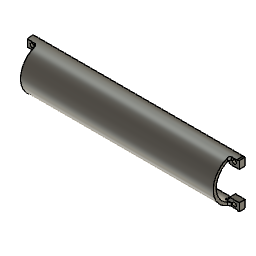
Cache cable (Autodesk Fusion 360 design; units mm, degrees)
Autodesk Fusion 360 part; units mm, degrees
sketch "Esquisse1" plane through (0, 0, 0) normal (1, 0, 0) x (0, 1, 0)
  circle A0 centre (0, 10) radius 10
  circle A1 centre (0, 10) radius 11.5
  line L0 (0, -1.5) -> (0, 21.5)
  dimension "d1" = 20
  dimension "d2" = 23
  constraint coincident origin A0
  constraint concentric A0 A1
  constraint coincident A1 L0.start
  constraint coincident A1 L0.end
  constraint vertical L0
  measures "d1" diameter of A0
  measures "d2" diameter of A1
extrude "Extrusion1" add sketch "Esquisse1" against normal blind 100 contours A0 A1 L0 picked at (-1.0681, 20.92)
sketch "Esquisse2" plane through (0, 0, 0) normal (0, 1, 0) x (1, 0, 0)
  line L0 (0, -21.5) -> (5, -21.5)
  line L1 (5, -21.5) -> (5, -17.5)
  line L2 (5, -17.5) -> (0, -17.5)
  line L3 (0, -17.5) -> (0, -21.5)
  line L4 (0, 1.5) -> (5, 1.5)
  line L5 (5, 1.5) -> (5, -2.5)
  line L6 (5, -2.5) -> (0, -2.5)
  line L7 (0, -2.5) -> (0, 1.5)
  circle A0 centre (2.5, -19.5) radius 1
  circle A1 centre (2.5, -0.5) radius 1
  line L8 (-100, -17.5) -> (-105, -17.5)
  line L9 (-105, -17.5) -> (-105, -21.5)
  line L10 (-105, -21.5) -> (-100, -21.5)
  line L11 (-100, -21.5) -> (-100, -17.5)
  line L12 (-100, 1.5) -> (-105, 1.5)
  line L13 (-105, 1.5) -> (-105, -2.5)
  line L14 (-105, -2.5) -> (-100, -2.5)
  line L15 (-100, -2.5) -> (-100, 1.5)
  circle A2 centre (-102.5, -19.5) radius 1
  circle A3 centre (-102.5, -0.5) radius 1
  dimension "d5" = 1.5
  dimension "d6" = 21.5
  dimension "d9" = 4
  dimension "d10" = 4
  dimension "d11" = 2
  dimension "d12" = 2
  dimension "d13" = 2.5
  dimension "d14" = 2
  dimension "d15" = 5
  dimension "d16" = 2.5
  dimension "d17" = 2
  dimension "d24" = 100
  dimension "d25" = 100
  dimension "d26" = 1.5
  dimension "d27" = 23
  dimension "d28" = 4
  dimension "d29" = 4
  dimension "d30" = 5
  dimension "d31" = 5
  dimension "d32" = 2
  dimension "d33" = 2
  dimension "d34" = 2.5
  dimension "d35" = 2
  dimension "d36" = 2.5
  dimension "d37" = 2
  constraint horizontal L0
  constraint vertical L1
  constraint horizontal L2
  constraint vertical L3
  constraint horizontal L4
  constraint vertical L5
  constraint horizontal L6
  constraint vertical L7
  constraint horizontal L8
  constraint vertical L9
  constraint horizontal L10
  constraint vertical L11
  constraint horizontal L12
  constraint vertical L13
  constraint horizontal L14
  constraint vertical L15
  measures "d5" distance of origin L4
  measures "d6" distance of origin L0
  measures "d9" distance of L4.end L5.end
  measures "d10" distance of L0.end L1.end
  measures "d11" diameter of A0
  measures "d12" diameter of A1
  measures "d13" distance of L5 A1.centre
  measures "d14" distance of L6 A1.centre
  measures "d15" distance of L4.start L5
  measures "d16" distance of L1 A0.centre
  measures "d17" vertical distance of L1.end A0.centre
  measures "d24" distance of origin L11
  measures "d25" distance of origin L15
  measures "d26" distance of origin L12
  measures "d27" distance of L10 L12
  measures "d28" distance of L8.end L9.end
  measures "d29" distance of L12.end L13.end
  measures "d30" distance of L9.end L10.end
  measures "d31" distance of L13.end L14.end
  measures "d32" diameter of A2
  measures "d33" distance of L10 A2.centre
  measures "d34" distance of L9 A2.centre
  measures "d35" diameter of A3
  measures "d36" distance of L13 A3.centre
  measures "d37" distance of L14 A3.centre
extrude "Extrusion2" add sketch "Esquisse2" against normal blind 3
fillet "Congé1" radius 2.5 1 edges at (0, -1.5176, 0.1158)
fillet "Congé2" radius 2.5 1 edges at (0, -1.5176, 19.8842)
fillet "Congé3" radius 1 2 edges at (0, -3, 20.3206) (0, -3, -0.3206)
fillet "Congé4" radius 2.5 1 edges at (-100, -1.5176, 19.8842)
fillet "Congé5" radius 2.5 1 edges at (-100, -1.5176, 0.1158)
fillet "Congé6" radius 1 2 edges at (-100, -3, 20.3206) (-100, -3, -0.3206)
sketch "Esquisse3" plane through (0, 0, 0) normal (1, 0, 0) x (0, 1, 0)
  circle A0 centre (0, 10) radius 11.5
  circle A1 centre (0, 10) radius 14.0357
  dimension "d44" = 10
  dimension "d45" = 23
  constraint concentric A0 A1
  measures "d44" distance of origin A0.centre
  measures "d45" diameter of A0
extrude "Extrusion3" cut sketch "Esquisse3" along normal blind -107 and the other way blind -4
